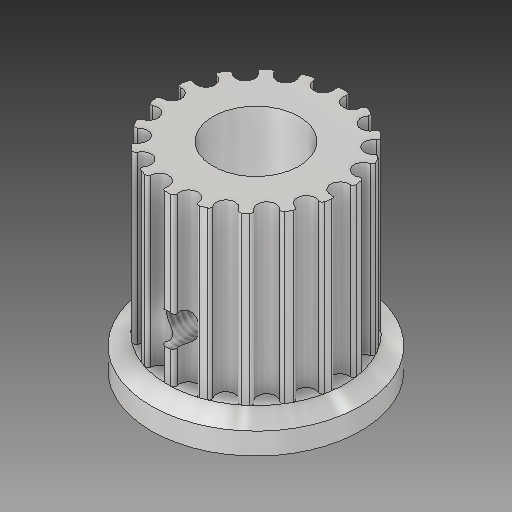
# Autodesk Inventor part: Motor Pulley
Saved by Autodesk Inventor 2019.3 (Build 233278000, 278)
## iProperties
Created: 2018-11-27
Part Number: Motor Pulley
Material: Aluminum 6061-AHC
Document SubType Name: Modeling
Designer: Petar
Density: 2.7 g/cm^3
Appearance: Aluminum - Dark
Mass: 7.08007 g
Surface Area: 23.296 cm^2
Volume: 2.62225 cm^3
Author: Petar
Autodesk Inventor part; units mm, degrees
ref_plane "YZ Plane" through (0, 0, 0) normal (1, 0, 0) x (0, 1, 0)
ref_plane "XZ Plane" through (0, 0, 0) normal (0, 1, 0) x (-1, 0, 0)
derived "gates_P18-3M-09AL.ipt"
sketch "Sketch1" plane through (8.2975, 9.8044, 4.3263) normal (0, 1, 0) x (1, 0, 0)
  circle A0 centre (-8.2975, 4.3263) radius 8.763
  arc A1 (-8.0454, 12.5394) -> (-8.614, 12.5371) centre (-8.2975, 4.3263) ccw
  arc A2 (-7.8093, 12.2146) -> (-8.0454, 12.5394) centre (-8.0532, 12.2855) ccw
  arc A3 (-7.8093, 12.2146) -> (-6.1179, 11.9232) centre (-6.98, 11.9735) ccw
  arc A4 (-5.7867, 12.1503) -> (-6.1179, 11.9232) centre (-5.8643, 11.9084) ccw
  arc A5 (-5.2516, 11.9579) -> (-5.7867, 12.1503) centre (-8.2975, 4.3263) ccw
  arc A6 (-5.1408, 11.5719) -> (-5.2516, 11.9579) centre (-5.3457, 11.722) ccw
  arc A7 (-5.1408, 11.5719) -> (-3.651, 10.7196) centre (-4.444, 11.0617) ccw
  arc A8 (-3.2622, 10.8197) -> (-3.651, 10.7196) centre (-3.4178, 10.619) ccw
  arc A9 (-2.8251, 10.4559) -> (-3.2622, 10.8197) centre (-8.2975, 4.3263) ccw
  arc A10 (-2.853, 10.0553) -> (-2.8251, 10.4559) centre (-2.9943, 10.2664) ccw
  arc A11 (-2.853, 10.0553) -> (-1.7446, 8.7449) centre (-2.3728, 9.3375) ccw
  arc A12 (-1.345, 8.7059) -> (-1.7446, 8.7449) centre (-1.5599, 8.5705) ccw
  arc A13 (-1.0587, 8.2146) -> (-1.345, 8.7059) centre (-8.2975, 4.3263) ccw
  arc A14 (-1.2219, 7.8477) -> (-1.0587, 8.2146) centre (-1.2825, 8.0944) ccw
  arc A15 (-1.2219, 7.8477) -> (-0.6286, 6.2372) centre (-1.0161, 7.009) ccw
  arc A16 (-0.2664, 6.0639) -> (-0.6286, 6.2372) centre (-0.5146, 6.0102) ccw
  arc A17 (-0.1654, 5.5043) -> (-0.2664, 6.0639) centre (-8.2975, 4.3263) ccw
  arc A18 (-0.4443, 5.2154) -> (-0.1654, 5.5043) centre (-0.4168, 5.4679) ccw
  arc A19 (-0.4443, 5.2154) -> (-0.4375, 3.4991) centre (-0.5378, 4.3568) ccw
  arc A20 (-0.1564, 3.2123) -> (-0.4375, 3.4991) centre (-0.4081, 3.2468) ccw
  arc A21 (-0.253, 2.6519) -> (-0.1564, 3.2123) centre (-8.2975, 4.3263) ccw
  arc A22 (-0.6138, 2.4758) -> (-0.253, 2.6519) centre (-0.5016, 2.7037) ccw
  arc A23 (-0.6138, 2.4758) -> (-1.1945, 0.8607) centre (-0.9953, 1.701) ccw
  arc A24 (-1.0284, 0.4951) -> (-1.1945, 0.8607) centre (-1.2531, 0.6136) ccw
  arc A25 (-1.3108, 0.0015) -> (-1.0284, 0.4951) centre (-8.2975, 4.3263) ccw
  arc A26 (-1.7101, -0.0406) -> (-1.3108, 0.0015) centre (-1.5268, 0.1352) ccw
  arc A27 (-1.7101, -0.0406) -> (-2.8082, -1.3596) centre (-2.3336, -0.6381) ccw
  arc A28 (-2.7771, -1.76) -> (-2.8082, -1.3596) centre (-2.9478, -1.5718) ccw
  arc A29 (-3.2113, -2.1272) -> (-2.7771, -1.76) centre (-8.2975, 4.3263) ccw
  arc A30 (-3.601, -2.0302) -> (-3.2113, -2.1272) centre (-3.3685, -1.9277) ccw
  arc A31 (-3.601, -2.0302) -> (-5.084, -2.8942) centre (-4.3912, -2.3785) ccw
  arc A32 (-5.1917, -3.281) -> (-5.084, -2.8942) centre (-5.2877, -3.0458) ccw
  arc A33 (-5.7253, -3.4776) -> (-5.1917, -3.281) centre (-8.2975, 4.3263) ccw
  arc A34 (-6.0583, -3.2531) -> (-5.7253, -3.4776) centre (-5.8048, -3.2364) ccw
  arc A35 (-6.0583, -3.2531) -> (-7.7473, -3.5578) centre (-6.92, -3.3102) ccw
  arc A36 (-7.9809, -3.8845) -> (-7.7473, -3.5578) centre (-7.9906, -3.6306) ccw
  arc A37 (-8.5495, -3.8867) -> (-7.9809, -3.8845) centre (-8.2975, 4.3263) ccw
  arc A38 (-8.7856, -3.5619) -> (-8.5495, -3.8867) centre (-8.5417, -3.6328) ccw
  arc A39 (-8.7856, -3.5619) -> (-10.477, -3.2705) centre (-9.6149, -3.3208) ccw
  arc A40 (-10.8082, -3.4976) -> (-10.477, -3.2705) centre (-10.7306, -3.2557) ccw
  arc A41 (-11.3434, -3.3052) -> (-10.8082, -3.4976) centre (-8.2975, 4.3263) ccw
  arc A42 (-11.4541, -2.9192) -> (-11.3434, -3.3052) centre (-11.2492, -3.0693) ccw
  arc A43 (-11.4541, -2.9192) -> (-12.9439, -2.0669) centre (-12.1509, -2.409) ccw
  arc A44 (-13.3327, -2.167) -> (-12.9439, -2.0669) centre (-13.1771, -1.9663) ccw
  arc A45 (-13.7698, -1.8032) -> (-13.3327, -2.167) centre (-8.2975, 4.3263) ccw
  arc A46 (-13.7419, -1.4026) -> (-13.7698, -1.8032) centre (-13.6006, -1.6137) ccw
  arc A47 (-13.7419, -1.4026) -> (-14.8503, -0.0922) centre (-14.2221, -0.6848) ccw
  arc A48 (-15.2499, -0.0532) -> (-14.8503, -0.0922) centre (-15.035, 0.0822) ccw
  arc A49 (-15.5362, 0.4381) -> (-15.2499, -0.0532) centre (-8.2975, 4.3263) ccw
  arc A50 (-15.373, 0.805) -> (-15.5362, 0.4381) centre (-15.3124, 0.5583) ccw
  arc A51 (-15.373, 0.805) -> (-15.9663, 2.4155) centre (-15.5788, 1.6437) ccw
  arc A52 (-16.3285, 2.5888) -> (-15.9663, 2.4155) centre (-16.0803, 2.6425) ccw
  arc A53 (-16.4295, 3.1484) -> (-16.3285, 2.5888) centre (-8.2975, 4.3263) ccw
  arc A54 (-16.1506, 3.4373) -> (-16.4295, 3.1484) centre (-16.1781, 3.1848) ccw
  arc A55 (-16.1506, 3.4373) -> (-16.1574, 5.1536) centre (-16.0572, 4.2959) ccw
  arc A56 (-16.4385, 5.4404) -> (-16.1574, 5.1536) centre (-16.1868, 5.4059) ccw
  arc A57 (-16.3419, 6.0008) -> (-16.4385, 5.4404) centre (-8.2975, 4.3263) ccw
  arc A58 (-15.9811, 6.1769) -> (-16.3419, 6.0008) centre (-16.0933, 5.949) ccw
  arc A59 (-15.9811, 6.1769) -> (-15.4004, 7.792) centre (-15.5996, 6.9517) ccw
  arc A60 (-15.5665, 8.1576) -> (-15.4004, 7.792) centre (-15.3418, 8.0391) ccw
  arc A61 (-15.2841, 8.6512) -> (-15.5665, 8.1576) centre (-8.2975, 4.3263) ccw
  arc A62 (-14.8848, 8.6932) -> (-15.2841, 8.6512) centre (-15.0681, 8.5175) ccw
  arc A63 (-14.8848, 8.6932) -> (-13.7867, 10.0123) centre (-14.2613, 9.2908) ccw
  arc A64 (-13.8178, 10.4127) -> (-13.7867, 10.0123) centre (-13.6471, 10.2245) ccw
  arc A65 (-13.3836, 10.7799) -> (-13.8178, 10.4127) centre (-8.2975, 4.3263) ccw
  arc A66 (-12.9939, 10.6829) -> (-13.3836, 10.7799) centre (-13.2264, 10.5804) ccw
  arc A67 (-12.9939, 10.6829) -> (-11.511, 11.5469) centre (-12.2037, 11.0312) ccw
  arc A68 (-11.4032, 11.9337) -> (-11.511, 11.5469) centre (-11.3072, 11.6985) ccw
  arc A69 (-10.8696, 12.1303) -> (-11.4032, 11.9337) centre (-8.2975, 4.3263) ccw
  arc A70 (-10.5366, 11.9058) -> (-10.8696, 12.1303) centre (-10.7901, 11.8891) ccw
  arc A71 (-10.5366, 11.9058) -> (-8.8476, 12.2105) centre (-9.6749, 11.9629) ccw
  arc A72 (-8.614, 12.5371) -> (-8.8476, 12.2105) centre (-8.6043, 12.2833) ccw
  point P0 (-8.2975, 4.3263)
sketch "Sketch2" plane through (0, 0, 0) normal (1, 0, 0) x (0, 1, 0)
  line L0 (0, 0) -> (13.436, 0) construction
  line L1 (0, -4) -> (13.436, -4)
  line L2 (13.436, 0) -> (13.436, -5.7717) construction
  line L3 (0, 0) -> (0, -9.7169) construction
  line L4 (3, -5.7717) -> (13.436, -5.7717)
  line L5 (0, -9.7169) -> (0, -4)
  line L6 (3, -5.7717) -> (3, -9.7169)
  line L7 (3, -9.7169) -> (0, -9.7169)
  line L8 (13.436, -4) -> (13.436, -5.7717)
  line L9 (13.436, -4.5717) -> (0, -4.5717) construction
  line L10 (9.8044, -8.2169) -> (9.8044, -8.2108) projected
  line L11 (9.8044, -7.2455) -> (9.8044, -5.8717) projected
  point P0 (9.8044, -8.213)
  point P1 (9.8044, -6.3932)
  dimension "d1" = 4
  dimension "d6" = 10.436
  dimension "d7" = 3
  dimension "d9" = 1.2
  dimension "d42" = 0.1
  dimension "d43" = 1.5
  constraints: 22 end point, 4 point on line, 3 horizontal, 3 vertical, 2 perpendicular, 1 collinear
  measures "d1" distance between parallel lines of L1 L0
  measures "d6" distance between parallel lines of L2 L6
  measures "d7" distance between parallel lines of L3 L6
  measures "d9" distance between parallel lines of L4 L9
  measures "d42" distance from line of L11.end L4
  measures "d43" distance from line of L10.start L7
revolve "Revolution1" add sketch "Sketch2" angle 360 about axis through (0, 0, 0) along (0, 1, 0)
ref_plane "Work Plane1" through (0, 18.436, 0) normal (0, 1, 0) x (1, 0, 0)
chamfer "Chamfer1" distance 1 distance2 1.5 1 edges at (0, 3, 9.7169) measured on face at (0, 2.5, 9.7169)
sketch "Sketch10" plane through (0, 18.436, 0) normal (0, 1, 0) x (1, 0, 0)
  arc A0 (3.1567, 7.2455) -> (4.6464, 6.3932) centre (3.8535, 6.7353) ccw projected
  arc A1 (0.4882, 7.8882) -> (2.1796, 7.5968) centre (1.3174, 7.6471) ccw projected
  arc A2 (-2.2392, 7.5795) -> (-0.5501, 7.8842) centre (-1.3775, 7.6365) ccw projected
  arc A3 (-4.6965, 6.3565) -> (-3.2135, 7.2205) centre (-3.9062, 6.7049) ccw projected
  arc A4 (-6.5873, 4.3669) -> (-5.4893, 5.686) centre (-5.9639, 4.9645) ccw projected
  arc A5 (-7.6836, 1.8505) -> (-7.1029, 3.4656) centre (-7.3022, 2.6253) ccw projected
  arc A6 (-7.8532, -0.889) -> (-7.8599, 0.8273) centre (-7.7597, -0.0305) ccw projected
  arc A7 (-7.0755, -3.5213) -> (-7.6688, -1.9109) centre (-7.2813, -2.6826) ccw projected
  arc A8 (-5.4444, -5.7289) -> (-6.5528, -4.4185) centre (-5.9247, -5.0112) ccw projected
  arc A9 (-3.1567, -7.2455) -> (-4.6464, -6.3932) centre (-3.8535, -6.7353) ccw projected
  arc A10 (-0.4882, -7.8882) -> (-2.1796, -7.5968) centre (-1.3174, -7.6471) ccw projected
  arc A11 (2.2392, -7.5795) -> (0.5501, -7.8842) centre (1.3775, -7.6365) ccw projected
  arc A12 (4.6965, -6.3565) -> (3.2135, -7.2205) centre (3.9062, -6.7049) ccw projected
  arc A13 (6.5873, -4.3669) -> (5.4893, -5.686) centre (5.9639, -4.9645) ccw projected
  arc A14 (7.6836, -1.8505) -> (7.1029, -3.4656) centre (7.3022, -2.6253) ccw projected
  arc A15 (7.8532, 0.889) -> (7.8599, -0.8273) centre (7.7597, 0.0305) ccw projected
  arc A16 (5.4444, 5.7289) -> (6.5528, 4.4185) centre (5.9247, 5.0112) ccw projected
  arc A17 (7.0755, 3.5213) -> (7.6688, 1.9109) centre (7.2813, 2.6826) ccw projected
  arc A18 (7.2387, 3.8882) -> (6.9525, 4.3796) centre (0, 0) ccw projected
  arc A19 (6.9525, 4.3796) -> (6.5528, 4.4185) centre (6.7375, 4.2442) ccw projected
  arc A20 (7.0755, 3.5213) -> (7.2387, 3.8882) centre (7.015, 3.768) ccw projected
  arc A21 (8.0311, 1.7376) -> (7.6688, 1.9109) centre (7.7828, 1.6839) ccw projected
  arc A22 (8.132, 1.1779) -> (8.0311, 1.7376) centre (0, 0) ccw projected
  arc A23 (7.8532, 0.889) -> (8.132, 1.1779) centre (7.8807, 1.1415) ccw projected
  arc A24 (8.141, -1.114) -> (7.8599, -0.8273) centre (7.8894, -1.0796) ccw projected
  arc A25 (8.0445, -1.6744) -> (8.141, -1.114) centre (0, 0) ccw projected
  arc A26 (7.6836, -1.8505) -> (8.0445, -1.6744) centre (7.7958, -1.6227) ccw projected
  arc A27 (7.2691, -3.8312) -> (7.1029, -3.4656) centre (7.0444, -3.7128) ccw projected
  arc A28 (6.9867, -4.3248) -> (7.2691, -3.8312) centre (0, 0) ccw projected
  arc A29 (6.5873, -4.3669) -> (6.9867, -4.3248) centre (6.7707, -4.1911) ccw projected
  arc A30 (5.5203, -6.0863) -> (5.4893, -5.686) centre (5.3497, -5.8982) ccw projected
  arc A31 (5.0861, -6.4536) -> (5.5203, -6.0863) centre (0, 0) ccw projected
  arc A32 (4.6965, -6.3565) -> (5.0861, -6.4536) centre (4.9289, -6.2541) ccw projected
  arc A33 (3.1058, -7.6073) -> (3.2135, -7.2205) centre (3.0098, -7.3722) ccw projected
  arc A34 (2.5721, -7.8039) -> (3.1058, -7.6073) centre (0, 0) ccw projected
  arc A35 (2.2392, -7.5795) -> (2.5721, -7.8039) centre (2.4926, -7.5627) ccw projected
  arc A36 (0.3166, -8.2108) -> (0.5501, -7.8842) centre (0.3068, -7.957) ccw projected
  arc A37 (-0.2521, -8.213) -> (0.3166, -8.2108) centre (0, 0) ccw projected
  arc A38 (-0.4882, -7.8882) -> (-0.2521, -8.213) centre (-0.2443, -7.9592) ccw projected
  arc A39 (-2.5108, -7.8239) -> (-2.1796, -7.5968) centre (-2.4331, -7.5821) ccw projected
  arc A40 (-3.0459, -7.6315) -> (-2.5108, -7.8239) centre (0, 0) ccw projected
  arc A41 (-3.1567, -7.2455) -> (-3.0459, -7.6315) centre (-2.9517, -7.3956) ccw projected
  arc A42 (-5.0353, -6.4933) -> (-4.6464, -6.3932) centre (-4.8796, -6.2926) ccw projected
  arc A43 (-5.4723, -6.1295) -> (-5.0353, -6.4933) centre (0, 0) ccw projected
  arc A44 (-5.4444, -5.7289) -> (-5.4723, -6.1295) centre (-5.3032, -5.94) ccw projected
  arc A45 (-6.9525, -4.3796) -> (-6.5528, -4.4185) centre (-6.7375, -4.2442) ccw projected
  arc A46 (-7.0755, -3.5213) -> (-7.2387, -3.8882) centre (-7.015, -3.768) ccw projected
  arc A47 (-7.2387, -3.8882) -> (-6.9525, -4.3796) centre (0, 0) ccw projected
  arc A48 (-8.0311, -1.7376) -> (-7.6688, -1.9109) centre (-7.7828, -1.6839) ccw projected
  arc A49 (-8.132, -1.1779) -> (-8.0311, -1.7376) centre (0, 0) ccw projected
  arc A50 (-7.8532, -0.889) -> (-8.132, -1.1779) centre (-7.8807, -1.1415) ccw projected
  arc A51 (-8.141, 1.114) -> (-7.8599, 0.8273) centre (-7.8894, 1.0796) ccw projected
  arc A52 (-8.0445, 1.6744) -> (-8.141, 1.114) centre (0, 0) ccw projected
  arc A53 (-7.6836, 1.8505) -> (-8.0445, 1.6744) centre (-7.7958, 1.6227) ccw projected
  arc A54 (-7.2691, 3.8312) -> (-7.1029, 3.4656) centre (-7.0444, 3.7128) ccw projected
  arc A55 (-6.9867, 4.3248) -> (-7.2691, 3.8312) centre (0, 0) ccw projected
  arc A56 (-6.5873, 4.3669) -> (-6.9867, 4.3248) centre (-6.7707, 4.1911) ccw projected
  arc A57 (-5.5203, 6.0863) -> (-5.4893, 5.686) centre (-5.3497, 5.8982) ccw projected
  arc A58 (-5.0861, 6.4536) -> (-5.5203, 6.0863) centre (0, 0) ccw projected
  arc A59 (-4.6965, 6.3565) -> (-5.0861, 6.4536) centre (-4.9289, 6.2541) ccw projected
  arc A60 (-3.1058, 7.6073) -> (-3.2135, 7.2205) centre (-3.0098, 7.3722) ccw projected
  arc A61 (-2.5721, 7.8039) -> (-3.1058, 7.6073) centre (0, 0) ccw projected
  arc A62 (-2.2392, 7.5795) -> (-2.5721, 7.8039) centre (-2.4926, 7.5627) ccw projected
  arc A63 (-0.3166, 8.2108) -> (-0.5501, 7.8842) centre (-0.3068, 7.957) ccw projected
  arc A64 (0.2521, 8.213) -> (-0.3166, 8.2108) centre (0, 0) ccw projected
  arc A65 (0.4882, 7.8882) -> (0.2521, 8.213) centre (0.2443, 7.9592) ccw projected
  arc A66 (2.5108, 7.8239) -> (2.1796, 7.5968) centre (2.4331, 7.5821) ccw projected
  arc A67 (3.0459, 7.6315) -> (2.5108, 7.8239) centre (0, 0) ccw projected
  arc A68 (3.1567, 7.2455) -> (3.0459, 7.6315) centre (2.9517, 7.3956) ccw projected
  arc A69 (5.0353, 6.4933) -> (4.6464, 6.3932) centre (4.8796, 6.2926) ccw projected
  arc A70 (5.4723, 6.1295) -> (5.0353, 6.4933) centre (0, 0) ccw projected
  arc A71 (5.4444, 5.7289) -> (5.4723, 6.1295) centre (5.3032, 5.94) ccw projected
  point P0 (0, 0)
extrude "Extrusion4" add sketch "Sketch10" against normal up to surface (15.436 mm away)
sketch "Sketch11" plane through (0, 0, 0) normal (0, -1, 0) x (1, 0, 0)
  circle A0 centre (0, 0) radius 4
  dimension "d48" = 8
  constraints: 1 centre point
  measures "d48" diameter of A0
sketch "Sketch7" plane through (0, 0, 0) normal (0, 0, 1) x (1, 0, 0)
  circle A0 centre (0, 7.436) radius 1.5
  line L0 (-4, 13.436) -> (4, 13.436) projected
  point P0 (0, 0)
  point P1 (0, 13.436)
  point P2 (0, 13.436)
  dimension "d26" = 3
  dimension "d37" = 6
  constraints: 1 centre point
  measures "d26" diameter of A0
  measures "d37" distance from line of L0 A0.centre
extrude "Extrusion3" cut sketch "Sketch7" along normal through all
thread "Thread1" size "M3x0.5" class "6H" standard "ANSI Metric M Profile" full length
extrude "Extrusion6" cut sketch "Sketch11" against normal through all
body "Solid1"
